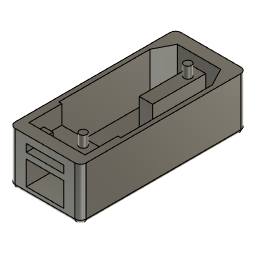
DHT22 case (Autodesk Fusion 360 design; units mm, degrees)
Autodesk Fusion 360 part; units mm, degrees
sketch "base" plane through (0, 0, 0) normal (0, 0, 1) x (1, 0, 0)
  line L0 (0, 0) -> (19, 0)
  line L1 (19, 0) -> (19, 44.4)
  line L2 (19, 44.4) -> (0, 44.4)
  line L3 (0, 44.4) -> (0, 0)
  dimension "d1" = 19
  dimension "d2" = 44.4
  constraint horizontal L0
  constraint vertical L1
  constraint horizontal L2
  constraint vertical L3
  constraint coincident L0.start L3.end
  measures "d1" distance of L0.start L0.end
  measures "d2" distance of L0.start L2.end
extrude "Extrude1" add sketch "base" along normal blind 2
sketch "walls" plane through (0, 0, 2) normal (0, 0, 1) x (-1, 0, 0)
  line L0 (0, -44.4) -> (0, 0)
  line L1 (0, 0) -> (-19, 0)
  line L2 (-19, 0) -> (-19, -44.4)
  line L3 (-19, -44.4) -> (0, -44.4)
  line L4 (0, 0) -> (-19, 0)
  line L5 (-19, 0) -> (-19, -44.4)
  line L6 (-19, -44.4) -> (0, -44.4)
  line L7 (0, -44.4) -> (0, 0)
  line L8 (-1.2, -12) -> (-17.8, -12)
  line L9 (-17.8, -12) -> (-17.8, -36.4)
  line L10 (-15.3, -41.2) -> (-3.7, -41.2)
  line L11 (-1.2, -36.4) -> (-1.2, -12)
  line L12 (-1.2, -36.4) -> (-3.7, -41.2)
  line L13 (-17.8, -36.4) -> (-15.3, -41.2)
  dimension "d5" = 19
  dimension "d6" = 44.4
  dimension "d7" = 16.6
  dimension "d9" = 12
  dimension "d10" = 1.2
  dimension "d59" = 4.8
  dimension "d61" = 4.8
  dimension "d62" = 2.5
  dimension "d63" = 11.6
  dimension "d64" = 3.2
  dimension "d71" = 2.5
  constraint horizontal L4
  constraint vertical L5
  constraint horizontal L6
  constraint vertical L7
  constraint coincident L0.end L1.start
  constraint horizontal L8
  constraint vertical L9
  constraint horizontal L10
  constraint vertical L11
  measures "d5" distance of L0.end L1.end
  measures "d6" distance of L0.end L0.start
  measures "d7" distance of L8.start L8.end
  measures "d9" distance of L4 L8
  measures "d10" distance of L7 L11
  measures "d59" distance of L10 L11.start
  measures "d61" distance of L10 L9.end
  measures "d62" distance of L9 L10.start
  measures "d63" distance of L10.end L10.start
  measures "d64" distance of L6 L10.end
  measures "d71" distance of L11 L10.end
extrude "Extrude2" add sketch "walls" along normal blind 12
sketch "hole for connector" plane through (0, 0, 0) normal (0, -1, 0) x (1, 0, 0)
  line L0 (0, 0) -> (19, 0)
  line L1 (19, 0) -> (19, 14)
  line L2 (19, 14) -> (0, 14)
  line L3 (0, 14) -> (0, 0)
  line L4 (0, 14) -> (19, 14) construction
  line L5 (19, 14) -> (19, 2) construction
  line L6 (19, 2) -> (0, 2) construction
  line L7 (0, 2) -> (0, 14) construction
  line L8 (9.5, 14) -> (9.5, 0) construction
  line L9 (4.5, 8.4) -> (14.5, 8.4)
  line L10 (14.5, 8.4) -> (14.5, 2)
  line L11 (14.5, 2) -> (4.5, 2)
  line L12 (4.5, 2) -> (4.5, 8.4)
  dimension "d13" = 10
  dimension "d14" = 6.4
  dimension "d15" = 2
  dimension "d16" = 4.5
  constraint horizontal L4
  constraint vertical L5
  constraint horizontal L6
  constraint vertical L7
  constraint coincident L1 L5.end
  constraint coincident L2.end L3.start
  constraint midpoint L2 L8.start
  constraint midpoint L0 L8.end
  constraint horizontal L9
  constraint vertical L10
  constraint horizontal L11
  constraint vertical L12
  measures "d13" distance of L9.start L9.end
  measures "d14" distance of L9.start L11.end
  measures "d15" distance of L0 L11
  measures "d16" distance of L7 L12
extrude "Extrude3" cut sketch "hole for connector" against normal blind 7 contours L9 L10 L11 L12
sketch "stand for rare of pcb" plane through (0, 0, 2) normal (0, 0, 1) x (-1, 0, 0)
  line L0 (-1.2, -12) -> (-17.8, -12)
  line L1 (-17.8, -12) -> (-17.8, -36.4)
  line L2 (-15.3, -41.2) -> (-3.7, -41.2)
  line L3 (-1.2, -36.4) -> (-1.2, -12)
  line L4 (-7.7, -41.2) -> (-11.3, -41.2)
  line L5 (-11.3, -41.2) -> (-11.3, -27)
  line L6 (-11.3, -27) -> (-7.7, -27)
  line L7 (-7.7, -27) -> (-7.7, -41.2)
  line L8 (-17.8, -12) -> (-1.2, -12)
  line L9 (-17.8, -36.4) -> (-15.3, -41.2)
  line L10 (-3.7, -41.2) -> (-1.2, -36.4)
  dimension "d27" = 3.6
  dimension "d28" = 15
  dimension "d29" = 6.5
  constraint horizontal L4
  constraint vertical L5
  constraint horizontal L6
  constraint vertical L7
  constraint coincident L2 L4.start
  measures "d27" distance of L4.start L4.end
  measures "d28" distance of L6 L8
  measures "d29" distance of L1 L5
extrude "Extrude5" add sketch "stand for rare of pcb" along normal blind 9 contours L2 L4 L5 L6 L7
sketch "hole for connector pins" plane through (0, 7, 0) normal (0, -1, 0) x (1, 0, 0)
  line L0 (4.5, 2) -> (14.5, 2)
  line L1 (14.5, 2) -> (14.5, 8.4)
  line L2 (14.5, 8.4) -> (4.5, 8.4)
  line L3 (4.5, 8.4) -> (4.5, 2)
  line L4 (5.5, 7.6) -> (13.5, 7.6)
  line L5 (13.5, 7.6) -> (13.5, 2)
  line L6 (13.5, 2) -> (5.5, 2)
  line L7 (5.5, 2) -> (5.5, 7.6)
  dimension "d32" = 8
  dimension "d33" = 5.6
  dimension "d34" = 5.5
  dimension "d35" = 2
  constraint horizontal L4
  constraint vertical L5
  constraint horizontal L6
  constraint vertical L7
  measures "d32" distance of L4.start L4.end
  measures "d33" distance of L4.start L6.end
  measures "d34" distance of origin L7
  measures "d35" distance of origin L6
extrude "Extrude6" cut sketch "hole for connector pins" against normal blind 5 contours L0 L4 L5 L6 L7
sketch "pit for pcb" plane through (0, 0, 14) normal (0, 0, 1) x (-1, 0, 0)
  line L0 (-1.2, -12) -> (-1.2, -36.4)
  line L1 (-3.7, -41.2) -> (-15.3, -41.2)
  line L2 (-17.8, -36.4) -> (-17.8, -12)
  line L3 (-17.8, -12) -> (-1.2, -12)
  line L4 (0, -44.4) -> (0, 0)
  line L5 (0, 0) -> (-19, 0)
  line L6 (-19, 0) -> (-19, -44.4)
  line L7 (-19, -44.4) -> (0, -44.4)
  line L8 (-2, -12) -> (-17, -12)
  line L9 (-17, -12) -> (-17, -3.2)
  line L10 (-17, -3.2) -> (-2, -3.2)
  line L11 (-2, -3.2) -> (-2, -12)
  line L12 (-1.2, -36.4) -> (-3.7, -41.2)
  line L13 (-15.3, -41.2) -> (-17.8, -36.4)
  dimension "d44" = 15
  dimension "d45" = 8.8
  dimension "d46" = 2
  dimension "d47" = 3.2
  constraint horizontal L8
  constraint vertical L9
  constraint horizontal L10
  constraint vertical L11
  measures "d44" distance of L8.start L8.end
  measures "d45" distance of L8.start L10.end
  measures "d46" distance of L4.end L11
  measures "d47" distance of L4.end L10
extrude "Extrude7" cut sketch "pit for pcb" against normal blind 3 contours L3 L8 L9 L10 L11
fillet "Fillet1" radius 1.5 4 edges at (19, 0, 7) (0, 0, 7) (0, 44.4, 7) (19, 44.4, 7)
sketch "pit for wires" plane through (0, 0, 11) normal (0, 0, 1) x (-1, 0, 0)
  line L0 (-2, -3.2) -> (-17, -3.2)
  line L1 (-17, -3.2) -> (-17, -12)
  line L2 (-2, -12) -> (-2, -3.2)
  line L3 (-4.5, -3.2) -> (-14.5, -3.2)
  line L4 (-14.5, -3.2) -> (-14.5, -7.2)
  line L5 (-4.5, -7.2) -> (-4.5, -3.2)
  line L6 (-2, -12) -> (-17, -12)
  line L7 (-17, -12) -> (-17, -7.2)
  line L8 (-2, -7.2) -> (-2, -12)
  line L9 (-17, -7.2) -> (-14.5, -7.2)
  line L10 (-4.5, -7.2) -> (-2, -7.2)
  line L11 (-17, -12) -> (-2, -12)
  dimension "d48" = 10
  dimension "d49" = 2.5
  dimension "d51" = 4
  dimension "d65" = 2.5
  constraint horizontal L3
  constraint vertical L4
  constraint vertical L5
  constraint coincident L0 L3.start
  constraint horizontal L6
  constraint vertical L7
  constraint horizontal L9
  constraint vertical L8
  constraint coincident L1 L7.end
  constraint coincident L2.start L6.start
  constraint collinear L9 L10
  measures "d48" distance of L3.start L3.end
  measures "d49" distance of L0.start L5
  measures "d51" distance of L0 L9
  measures "d65" distance of L1 L4
extrude "Extrude8" cut sketch "pit for wires" against normal blind 2 contours L0 L1 L2 L3 L4 L5 L6 L7 L8 L9 L10 L11
sketch "mount cylinder" plane through (0, 0, 11) normal (0, 0, 1) x (-1, 0, 0)
  line L0 (-7.7, -27) -> (-11.3, -27)
  line L1 (-11.3, -27) -> (-11.3, -41.2)
  line L2 (-11.3, -41.2) -> (-7.7, -41.2)
  line L3 (-7.7, -41.2) -> (-7.7, -27)
  circle A0 centre (-9.5, -38.2) radius 1
  line L4 (-17.8, -36.4) -> (-17.8, -12)
  dimension "d54" = 2
  dimension "d55" = 3
  dimension "d56" = 8.3
  measures "d54" diameter of A0
  measures "d55" distance of L2 A0.centre
  measures "d56" distance of A0.centre L4
extrude "Extrude9" add sketch "mount cylinder" along normal blind 3 contours A0
sketch "mount cylinder 2" plane through (0, 0, 9) normal (0, 0, 1) x (-1, 0, 0)
  line L0 (-14.5, -3.2) -> (-14.5, -7.2)
  line L1 (-14.5, -7.2) -> (-17, -7.2)
  line L2 (-17, -7.2) -> (-17, -12)
  line L3 (-17, -12) -> (-2, -12)
  line L4 (-2, -12) -> (-2, -7.2)
  line L5 (-2, -7.2) -> (-4.5, -7.2)
  line L6 (-4.5, -7.2) -> (-4.5, -3.2)
  circle A0 centre (-9.5, -10.2) radius 1
  line L7 (-4.5, -3.2) -> (-14.5, -3.2)
  dimension "d66" = 2
  dimension "d68" = 7.5
  dimension "d72" = 7
  measures "d66" diameter of A0
  measures "d68" distance of L2 A0.centre
  measures "d72" distance of A0.centre L7
extrude "Extrude10" add sketch "mount cylinder 2" along normal blind 3 contours A0
sketch "lock notch front" plane through (0, 0, 0) normal (0, -1, 0) x (1, 0, 0)
  line L0 (14.5, 8.4) -> (14.5, 2)
  line L1 (14.5, 2) -> (4.5, 2)
  line L2 (4.5, 2) -> (4.5, 8.4)
  line L3 (4.5, 8.4) -> (14.5, 8.4)
  line L4 (1.5, 14) -> (1.5, 0)
  line L5 (1.5, 0) -> (17.5, 0)
  line L6 (17.5, 0) -> (17.5, 14)
  line L7 (17.5, 14) -> (1.5, 14)
  line L8 (4.5, 12) -> (14.5, 12)
  line L9 (14.5, 12) -> (14.5, 10)
  line L10 (14.5, 10) -> (4.5, 10)
  line L11 (4.5, 10) -> (4.5, 12)
  dimension "d81" = 10
  dimension "d82" = 2
  dimension "d83" = 2
  dimension "d84" = 4.5
  constraint horizontal L8
  constraint vertical L9
  constraint horizontal L10
  constraint vertical L11
  measures "d81" distance of L8.start L8.end
  measures "d82" distance of L8.start L10.end
  measures "d83" distance of L7 L8
  measures "d84" distance of origin L11
sketch "lock notch back" plane through (0, 44.4, 0) normal (0, 1, 0) x (-1, 0, 0)
  line L0 (-17.5, 14) -> (-17.5, 0)
  line L1 (-17.5, 0) -> (-1.5, 0)
  line L2 (-1.5, 0) -> (-1.5, 14)
  line L3 (-1.5, 14) -> (-17.5, 14)
  line L4 (-14.5, 12) -> (-4.5, 12)
  line L5 (-4.5, 12) -> (-4.5, 10)
  line L6 (-4.5, 10) -> (-14.5, 10)
  line L7 (-14.5, 10) -> (-14.5, 12)
  dimension "d85" = 10
  dimension "d86" = 2
  dimension "d87" = 2
  dimension "d88" = 4.5
  constraint horizontal L4
  constraint vertical L5
  constraint horizontal L6
  constraint vertical L7
  measures "d85" distance of L4.start L4.end
  measures "d86" distance of L4.start L6.end
  measures "d87" distance of L3 L4
  measures "d88" distance of origin L5
extrude "Extrude12" cut sketch "lock notch back" against normal blind 2 contours L4 L5 L6 L7
extrude "Extrude13" cut sketch "lock notch front" against normal blind 2 contours L8 L9 L10 L11
fillet "Fillet2" radius 1 1 faces at (6.3333, 29.1, 0)
named bodies: "case"
